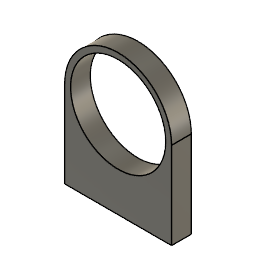
Thrust Bearing Worm (Autodesk Fusion 360 design; units mm, degrees)
part number: 2026-05-12-22-49-02-763
Autodesk Fusion 360 part; units mm, degrees
sketch "Sketch1" plane through (0, 0, 0) normal (0, 1, 0) x (1, 0, 0)
  line L0 (-10, 0) -> (17, 0)
  line L1 (17, 0) -> (17, -21.946)
  line L2 (17, -21.946) -> (-10, -21.946)
  line L3 (-10, -21.946) -> (-10, 0)
  dimension "d1" = 21.946
  dimension "d2" = 27
  dimension "d3" = 10
  dimension "d4" = 21.946
  constraint horizontal L0
  constraint vertical L1
  constraint horizontal L2
  constraint vertical L3
  measures "d1" distance of L0.start L2.end
  measures "d2" distance of L0.start L0.end
  measures "d3" distance of origin L0.start
  measures "d4" distance of origin L2
extrude "Extrude1" add sketch "Sketch1" along normal blind 5
sketch "Sketch2" plane through (0, 0, 0) normal (0, -1, 0) x (1, 0, 0)
  line L0 (17, 21.946) -> (-10, 21.946)
  line L1 (-10, 21.946) -> (-10, 0)
  line L2 (-10, 0) -> (17, 0)
  line L3 (17, 0) -> (17, 21.946)
  circle A0 centre (3.5, 21.946) radius 13.5
  circle A1 centre (3.5, 21.946) radius 12
  dimension "d7" = 27
  dimension "d8" = 24
  constraint midpoint L0 A0.centre
  constraint concentric A0 A1
  measures "d7" diameter of A0
  measures "d8" diameter of A1
extrude "Extrude2" add sketch "Sketch2" against normal blind 5 contours L0 A0 A1 picked at (13.449, 30.2624)
extrude "Extrude3" cut sketch "Sketch2" against normal blind 5 contours L0 A1 picked at (6.689, 16.5654)
equation "d1 = 21.616 mm + 0.33 mm"
equation "d4 = 21.616 mm + 0.33 mm"
